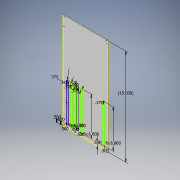
# Autodesk Inventor part: GlyphPlateUnderside
Saved by Autodesk Inventor 2017 (Build 210142000, 142)
## iProperties
Created: 2018-01-27
Part Number: GlyphPlateUnderside
Material: Generic
Document SubType Name: Modeling
Designer: User
Density: 1 g/cm^3
Appearance: Default
Author: User
Autodesk Inventor part; units mm, degrees
ref_plane "YZ Plane" through (0, 0, 0) normal (1, 0, 0) x (0, 1, 0)
ref_plane "XZ Plane" through (0, 0, 0) normal (0, 1, 0) x (-1, 0, 0)
ref_plane "XY Plane" through (0, 0, 0) normal (0, 0, 1) x (1, 0, 0)
sketch "Sketch1" plane through (0, 0, 0) normal (0, 0, 1) x (1, 0, 0)
  line L0 (0, 0) -> (178.2064, 0)
  line L1 (178.2064, 0) -> (178.2064, 381)
  line L2 (178.2064, 381) -> (0, 381)
  line L3 (0, 381) -> (0, 0)
  dimension "d0" = 178.2064
  dimension "d1" = 381
  constraints: 8 end point, 2 parallel, 1 horizontal, 1 perpendicular
  measures "d0" distance of L2.end L1.end
  measures "d1" distance of L1.end L0.end
extrude "Extrusion1" add sketch "Sketch1" along normal blind 3.175
sketch "Sketch2" plane through (0, 0, 3.175) normal (0, 0, 1) x (1, 0, 0)
  line L0 (0, 0) -> (178.2064, 0) projected
  line L1 (0, 0) -> (4.0386, 0)
  line L2 (4.0386, 0) -> (4.0386, 6.35)
  line L3 (0, 381) -> (0, 0) projected
  line L4 (0, 381) -> (4.0386, 381)
  line L5 (178.2064, 381) -> (0, 381) projected
  line L6 (4.0386, 381) -> (4.0386, 342.9)
  line L7 (4.0386, 381) -> (42.1386, 381) construction
  line L8 (0, 381) -> (0, 377.825)
  line L9 (0, 377.825) -> (6.35, 377.825)
  line L10 (178.2064, 0) -> (178.2064, 381) projected
  line L11 (178.2064, 0) -> (175.0314, 0)
  line L12 (175.0314, 0) -> (175.0314, 6.35)
  line L13 (178.2064, 377.825) -> (171.8564, 377.825)
  point P0 (175.0314, 368.3)
  dimension "d4" = 4.0386
  dimension "d5" = 6.35
  dimension "d6" = 38.1
  dimension "d7" = 90
  dimension "d8" = 3.175
  dimension "d9" = 6.35
  dimension "d10" = 3.175
  dimension "d11" = 6.35
  dimension "d19" = 4.0386
  dimension "d21" = 3.175
  dimension "d22" = 12.7
  dimension "d23" = 3.175
  constraints: 20 end point, 5 coincident, 5 perpendicular, 5 point on line, 1 horizontal, 1 vertical
  measures "d4" distance of L0.start L1.end
  measures "d5" distance of L1.end L2.end
  measures "d6" distance of L4.end L6.end
  measures "d7" angle of L6 L7
  measures "d8" distance of L3.start L8.end
  measures "d9" distance of L8.end L9.end
  measures "d10" distance of L0.end L11.end
  measures "d11" distance of L13.start L13.end
  measures "d19" distance between parallel lines of L3 L6
  measures "d21" distance from line of L10 point (175.031, 368.3)
  measures "d22" distance from line of point (175.031, 368.3) L5
  measures "d23" distance from line of L5 L13.end
hole "Hole1" at (4.0386, 6.35, 3.175) at (4.0386, 342.9, 3.175) at (6.35, 377.825, 3.175) at (175.0314, 6.35, 3.175) at (175.0314, 368.3, 3.175) at (171.8564, 377.825, 3.175) direction (0, 0, -1) diameter 3.556 depth 25.4 tip angle 118
sketch "Sketch3" plane through (0, 0, 3.175) normal (0, 0, 1) x (1, 0, 0)
  line L0 (17.4625, 12.7) -> (17.4625, 165.1) construction
  line L1 (22.225, 17.4625) -> (22.225, 160.3375)
  line L2 (12.7, 160.3375) -> (12.7, 17.4625)
  arc A0 (12.7, 17.4625) -> (22.225, 17.4625) centre (17.4625, 17.4625) ccw
  arc A1 (22.225, 160.3375) -> (12.7, 160.3375) centre (17.4625, 160.3375) ccw
  line L3 (33.6679, 12.7) -> (33.6679, 165.1) construction
  line L4 (38.4304, 17.4625) -> (38.4304, 160.3375)
  line L5 (28.9054, 160.3375) -> (28.9054, 17.4625)
  arc A2 (28.9054, 17.4625) -> (38.4304, 17.4625) centre (33.6679, 17.4625) ccw
  arc A3 (38.4304, 160.3375) -> (28.9054, 160.3375) centre (33.6679, 160.3375) ccw
  line L6 (160.7439, 12.7) -> (160.7439, 165.1) construction
  line L7 (165.5064, 17.4625) -> (165.5064, 160.3375)
  line L8 (155.9814, 160.3375) -> (155.9814, 17.4625)
  arc A4 (155.9814, 17.4625) -> (165.5064, 17.4625) centre (160.7439, 17.4625) ccw
  arc A5 (165.5064, 160.3375) -> (155.9814, 160.3375) centre (160.7439, 160.3375) ccw
  line L9 (0, 381) -> (0, 0) projected
  line L10 (178.2064, 0) -> (178.2064, 381) projected
  line L11 (47.9651, 12.7) -> (47.9651, 165.1) construction
  line L12 (52.7276, 17.4625) -> (52.7276, 160.3375)
  line L13 (43.2026, 160.3375) -> (43.2026, 17.4625)
  arc A6 (43.2026, 17.4625) -> (52.7276, 17.4625) centre (47.9651, 17.4625) ccw
  arc A7 (52.7276, 160.3375) -> (43.2026, 160.3375) centre (47.9651, 160.3375) ccw
  line L14 (73.7973, 12.7) -> (73.7973, 165.1) construction
  line L15 (78.5598, 17.4625) -> (78.5598, 160.3375)
  line L16 (69.0348, 160.3375) -> (69.0348, 17.4625)
  arc A8 (69.0348, 17.4625) -> (78.5598, 17.4625) centre (73.7973, 17.4625) ccw
  arc A9 (78.5598, 160.3375) -> (69.0348, 160.3375) centre (73.7973, 160.3375) ccw
  line L17 (0, 0) -> (178.2064, 0) projected
  point P0 (17.4625, 88.9)
  point P1 (33.6679, 88.9)
  point P2 (160.7439, 88.9)
  point P3 (47.9651, 88.9)
  point P4 (73.7973, 88.9)
  dimension "d24" = 9.525
  dimension "d25" = 9.525
  dimension "d26" = 9.525
  dimension "d27" = 12.7
  dimension "d28" = 12.7
  dimension "d30" = 9.525
  dimension "d31" = 0
  dimension "d32" = 0
  dimension "d33" = 9.525
  dimension "d34" = 12.7
  dimension "d35" = 12.7
  dimension "d36" = 12.7
  dimension "d37" = 12.7
  dimension "d39" = 381
  dimension "d40" = 152.4
  dimension "d41" = 152.4
  dimension "d42" = 152.4
  dimension "d43" = 152.4
  constraints: 40 end point, 30 point on circle, 20 tangent, 10 centre point, 10 point on line, 6 parallel, 5 midpoint, 4 vertical
  measures "d24" diameter of A1
  measures "d25" diameter of A3
  measures "d26" diameter of A5
  measures "d27" distance between parallel lines of L9 L2
  measures "d28" distance between parallel lines of L10 L7
  measures "d30" diameter of A7
  measures "d31" vertical distance of L11.end L3.end
  measures "d32" vertical distance of L11.start L3.start
  measures "d33" diameter of A9
  measures "d34" distance from line of L17 L0.start
  measures "d35" distance from line of L17 L3.start
  measures "d36" distance from line of L17 L14.start
  measures "d37" distance from line of L17 L6.start
  measures "d39" distance of L10.start L10.end
  measures "d40" distance of L11.start L11.end
  measures "d41" distance of L0.start L0.end
  measures "d42" distance of L14.start L14.end
  measures "d43" distance of L6.start L6.end
equation "\"d41\" = d40"
equation "\"d42\" = d40"
equation "\"d43\" = d40"
body "Solid1"
